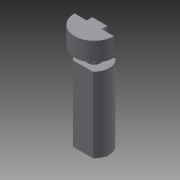
# Autodesk Inventor part: 308-106
Saved by Autodesk Inventor 2015 SP2 (Build 190223200, 223)
## iProperties
Created: 2016-07-20
Part Number: 308-106
Material: Generic
Document SubType Name: Modeling
Designer: Iain
Density: 1 g/cm^3
Appearance: Default
Author: Iain
Autodesk Inventor part; units mm, degrees
ref_plane "YZ Plane" through (0, 0, 0) normal (1, 0, 0) x (0, 1, 0)
ref_plane "XZ Plane" through (0, 0, 0) normal (0, 1, 0) x (-1, 0, 0)
ref_plane "XY Plane" through (0, 0, 0) normal (0, 0, 1) x (1, 0, 0)
sketch "Sketch2" plane through (0, 0, 0) normal (0, 0, 1) x (1, 0, 0)
  circle A0 centre (0, 0) radius 4
  dimension "d0" = 8
  constraints: 1 centre point, 1 coincident
  measures "d0" diameter of A0
extrude "Extrusion1" add sketch "Sketch2" against normal blind 20
sketch "Sketch3" plane through (0, 0, 0) normal (0, 0, 1) x (1, 0, 0)
  circle A0 centre (0, 0) radius 4 projected
  line L0 (-4, 3) -> (4, 3)
  line L1 (4, 3) -> (4, -3)
  line L2 (4, -3) -> (-4, -3)
  line L3 (-4, -3) -> (-4, 3)
  line L4 (-4, 3) -> (4, 3)
  line L5 (4, 3) -> (4, 4)
  line L6 (4, 4) -> (-4, 4)
  line L7 (-4, 4) -> (-4, 3)
  line L8 (-4, 0) -> (4, 0) construction
  point P0 (4, 3.5)
  dimension "d3" = 6
  constraints: 18 end point, 4 parallel, 3 horizontal, 3 midpoint, 3 tangent, 2 perpendicular, 1 horizontal alignment, 1 vertical alignment
  measures "d3" distance of L2.end L0.start
extrude "Extrusion2" cut sketch "Sketch3" against normal up to surface (20 mm away) from surface at 0 contours L0 A0 | A0 L6 L5 L0 | A0 L0 L7 L6
mirror "Mirror1" about plane through (0, 0, 0) normal (0, 1, 0) of "Extrusion2"
sketch "Sketch5" plane through (0, 0, 0) normal (0, 0, 1) x (1, 0, 0)
  circle A0 centre (0, 0) radius 1.75
  dimension "d6" = 3.5
  constraints: 1 centre point, 1 coincident
  measures "d6" diameter of A0
extrude "Extrusion3" add sketch "Sketch5" along normal blind 0.5
sketch "Sketch6" plane through (0, 0, 0) normal (0, 0, 1) x (1, 0, 0)
  circle A0 centre (0, 0) radius 0.5
  dimension "d9" = 1
  constraints: 1 centre point, 1 coincident
  measures "d9" diameter of A0
extrude "Extrusion4" add sketch "Sketch6" along normal blind 8
sketch "Sketch7" plane through (0, 0, 8) normal (0, 0, 1) x (1, 0, 0)
  circle A0 centre (0, 0) radius 5.25
  dimension "d12" = 10.5
  constraints: 1 centre point, 1 coincident
  measures "d12" diameter of A0
extrude "Extrusion5" add sketch "Sketch7" against normal blind 5
sketch "Sketch8" plane through (0, 0, 8) normal (0, 0, 1) x (1, 0, 0)
  circle A0 centre (0, 0) radius 5.25 projected
  line L0 (-2, 1.5) -> (2, 1.5)
  line L1 (2, 1.5) -> (2, 0)
  line L2 (2, 0) -> (-2, 0)
  line L3 (-2, 0) -> (-2, 1.5)
  line L4 (-5.25, 0) -> (5.25, 0)
  dimension "d15" = 4
  dimension "d16" = 1.5
  constraints: 10 end point, 3 coincident, 2 horizontal, 2 midpoint, 2 parallel, 2 point on circle, 1 perpendicular
  measures "d15" distance of L0.start L0.end
  measures "d16" distance of L2.end L0.start
extrude "Extrusion6" cut sketch "Sketch8" against normal up to surface (5 mm away) contours L4 L1 L0 L3 A0
sketch "Sketch9" plane through (0, 0, -20) normal (0, 0, -1) x (-1, 0, 0)
  circle A0 centre (0, 0) radius 1.75
  dimension "d19" = 3.5
  constraints: 1 centre point, 1 coincident
  measures "d19" diameter of A0
extrude "Extrusion7" add sketch "Sketch9" along normal blind 1
sketch "Sketch10" plane through (0, 0, -20) normal (0, 0, -1) x (-1, 0, 0)
  circle A0 centre (0, 0) radius 1.75 projected
  line L0 (-2.6458, -3) -> (2.6458, -3) projected
  arc A1 (2.6458, -3) -> (2.6458, 3) centre (0, 0) ccw projected
  line L1 (2.6458, 3) -> (-2.6458, 3) projected
  arc A2 (-2.6458, 3) -> (-2.6458, -3) centre (0, 0) ccw projected
  arc A3 (-2.6458, 3) -> (-2.6458, -3) centre (0, 0) ccw construction
  line L2 (-4, 0) -> (4, 0) construction
  arc A4 (2.6458, -3) -> (2.6458, 3) centre (0, 0) ccw construction
  line L3 (-3.9392, 0.6946) -> (3.9392, -0.6946) construction
  line L4 (-3.0153, 1.0394) -> (-2.7199, 0.9873)
  line L5 (-2.7199, 0.9873) -> (-2.8935, 0.0025)
  line L6 (-2.8935, 0.0025) -> (-3.189, 0.0546)
  line L7 (-3.189, 0.0546) -> (-3.0153, 1.0394)
  line L8 (0.3039, 1.7234) -> (-0.3039, -1.7234) construction
  line L9 (3.189, -0.0546) -> (2.8935, -0.0025)
  line L10 (2.8935, -0.0025) -> (2.7199, -0.9873)
  line L11 (2.7199, -0.9873) -> (3.0153, -1.0394)
  line L12 (3.0153, -1.0394) -> (3.189, -0.0546)
  point P0 (0, 0)
  dimension "d22" = 10
  dimension "d23" = 0.3
  dimension "d24" = 1
  dimension "d25" = 0.5
  dimension "d26" = 2.85
  constraints: 22 end point, 8 point on circle, 4 symmetric about line, 3 midpoint, 3 perpendicular, 2 parallel, 1 coincident
  measures "d22" angle of L2 L3
  measures "d23" distance of L4.start L4.end
  measures "d24" distance of L6.end L4.start
  measures "d25" distance between parallel lines of L3 L4
  measures "d26" distance from line of point (0, 0) L5
extrude "Extrusion8" add sketch "Sketch10" along normal blind 1 contours L4 L5 L6 L7 | L12 L11 L10 L9
ref_plane "Work Plane1" through (0, 0, 0) normal (0, 1, 0) x (-1, 0, 0)
equation "\"d25\" = 0.5 * d24"
body "Solid1"
